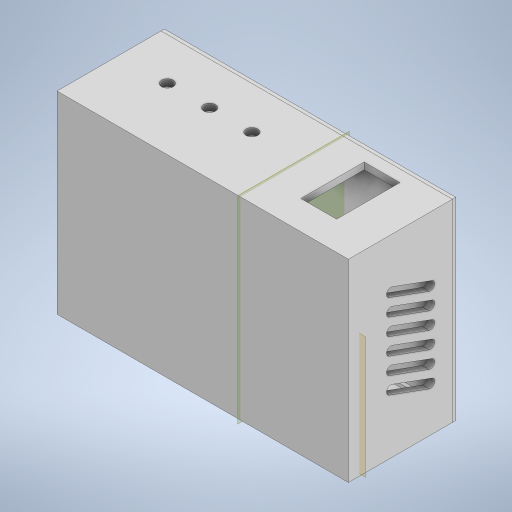
# Autodesk Inventor part: obudowa_attocube
Saved by Autodesk Inventor 2024 (Build 280153000, 153)
## iProperties
Created: 2025-11-29
Part Number: obudowa_attocube
Material: Generic
Document SubType Name: Modeling
Designer: tkazi
Density: 1 g/cm^3
Appearance: Default
Author: tkazi
Autodesk Inventor part; units mm, degrees
ref_plane "YZ Plane" through (0, 0, 0) normal (1, 0, 0) x (0, 1, 0)
ref_plane "XZ Plane" through (0, 0, 0) normal (0, 1, 0) x (-1, 0, 0)
ref_plane "XY Plane" through (0, 0, 0) normal (0, 0, 1) x (1, 0, 0)
ref_plane "Work Plane1" through (0, 0, 0) normal (0, 0, 1) x (1, 0, 0)
sketch "Sketch1" plane through (0, 0, 0) normal (0, 0, 1) x (1, 0, 0)
  line L0 (-218.6, -123.6) -> (-55.2, -123.6) projected
  line L1 (-55.2, -123.6) -> (-55.2, -58.2) projected
  line L2 (-55.2, -58.2) -> (-218.6, -58.2) projected
  line L3 (-218.6, -58.2) -> (-218.6, -123.6) projected
  circle A0 centre (-61.32, -115.13) radius 1.005 projected
  circle A1 centre (-71.48, -115.13) radius 1.005 projected
  circle A2 centre (-81.8, -118.4) radius 1.6 projected
  circle A3 centre (-91.52, -115.13) radius 1.005 projected
  circle A4 centre (-66.4, -110.05) radius 0.445 projected
  circle A5 centre (-68.94, -110.05) radius 0.445 projected
  circle A6 centre (-77.08, -109.65) radius 0.55 projected
  circle A7 centre (-77.08, -107.11) radius 0.55 projected
  circle A8 centre (-96.6, -110.05) radius 0.445 projected
  circle A9 centre (-99.14, -110.05) radius 0.445 projected
  circle A10 centre (-101.68, -115.13) radius 1.005 projected
  circle A11 centre (-121.72, -115.13) radius 1.005 projected
  circle A12 centre (-131.88, -115.13) radius 1.005 projected
  circle A13 centre (-107.28, -109.65) radius 0.55 projected
  circle A14 centre (-107.28, -107.11) radius 0.55 projected
  circle A15 centre (-126.8, -110.05) radius 0.445 projected
  circle A16 centre (-129.34, -110.05) radius 0.445 projected
  circle A17 centre (-137.48, -109.65) radius 0.55 projected
  circle A18 centre (-137.48, -107.11) radius 0.55 projected
  circle A19 centre (-77.08, -104.57) radius 0.55 projected
  circle A20 centre (-77.08, -96.83) radius 0.55 projected
  circle A21 centre (-77.08, -94.29) radius 0.55 projected
  circle A22 centre (-77.08, -91.75) radius 0.55 projected
  circle A23 centre (-107.28, -104.57) radius 0.55 projected
  circle A24 centre (-137.48, -104.57) radius 0.55 projected
  circle A25 centre (-107.28, -96.83) radius 0.55 projected
  circle A26 centre (-107.28, -94.29) radius 0.55 projected
  circle A27 centre (-107.28, -91.75) radius 0.55 projected
  circle A28 centre (-137.48, -96.83) radius 0.55 projected
  circle A29 centre (-137.48, -94.29) radius 0.55 projected
  circle A30 centre (-137.48, -91.75) radius 0.55 projected
  circle A31 centre (-159.11, -115.13) radius 0.51 projected
  circle A32 centre (-165.275, -115) radius 0.9 projected
  circle A33 centre (-170.725, -115) radius 0.9 projected
  circle A34 centre (-176.89, -115.13) radius 0.51 projected
  circle A35 centre (-159.11, -112.59) radius 0.51 projected
  circle A36 centre (-165.575, -111.97) radius 0.75 projected
  circle A37 centre (-159.11, -110.05) radius 0.51 projected
  circle A38 centre (-170.425, -111.97) radius 0.75 projected
  circle A39 centre (-176.89, -112.59) radius 0.51 projected
  circle A40 centre (-176.89, -110.05) radius 0.51 projected
  circle A41 centre (-159.11, -107.51) radius 0.51 projected
  circle A42 centre (-176.89, -107.51) radius 0.51 projected
  circle A43 centre (-190.29, -115.61) radius 0.4 projected
  circle A44 centre (-195.29, -115.61) radius 0.4 projected
  circle A45 centre (-203.8, -119.8) radius 0.8 projected
  arc A46 (-199.8, -118.55) -> (-198.8, -118.55) centre (-199.3, -118.55) ccw projected
  line L4 (-199.8, -117.05) -> (-199.8, -118.55) projected
  arc A47 (-198.8, -117.05) -> (-199.8, -117.05) centre (-199.3, -117.05) ccw projected
  line L5 (-198.8, -118.55) -> (-198.8, -117.05) projected
  arc A48 (-208.8, -118.55) -> (-207.8, -118.55) centre (-208.3, -118.55) ccw projected
  line L6 (-208.8, -117.05) -> (-208.8, -118.55) projected
  arc A49 (-207.8, -117.05) -> (-208.8, -117.05) centre (-208.3, -117.05) ccw projected
  line L7 (-207.8, -118.55) -> (-207.8, -117.05) projected
  arc A50 (-204.45, -116.3) -> (-204.45, -117.3) centre (-204.45, -116.8) ccw projected
  line L8 (-203.15, -116.3) -> (-204.45, -116.3) projected
  arc A51 (-203.15, -117.3) -> (-203.15, -116.3) centre (-203.15, -116.8) ccw projected
  line L9 (-204.45, -117.3) -> (-203.15, -117.3) projected
  circle A52 centre (-214.4, -115.8) radius 1.6 projected
  circle A53 centre (-188.555, -108.845) radius 0.55 projected
  circle A54 centre (-191.095, -108.845) radius 0.55 projected
  circle A55 centre (-193.635, -108.845) radius 0.55 projected
  arc A56 (-204.8, -110.3) -> (-204.8, -111.3) centre (-204.8, -110.8) ccw projected
  line L10 (-202.8, -110.3) -> (-204.8, -110.3) projected
  arc A57 (-202.8, -111.3) -> (-202.8, -110.3) centre (-202.8, -110.8) ccw projected
  line L11 (-204.8, -111.3) -> (-202.8, -111.3) projected
  circle A58 centre (-214.2, -109.2) radius 0.3 projected
  circle A59 centre (-159.11, -104.97) radius 0.51 projected
  circle A60 centre (-176.89, -104.97) radius 0.51 projected
  circle A61 centre (-159.11, -102.43) radius 0.51 projected
  circle A62 centre (-159.11, -99.89) radius 0.51 projected
  circle A63 centre (-176.89, -102.43) radius 0.51 projected
  circle A64 centre (-176.89, -99.89) radius 0.51 projected
  circle A65 centre (-159.11, -97.35) radius 0.51 projected
  circle A66 centre (-176.89, -97.35) radius 0.51 projected
  circle A67 centre (-159.11, -94.81) radius 0.51 projected
  circle A68 centre (-159.11, -92.27) radius 0.51 projected
  circle A69 centre (-176.89, -94.81) radius 0.51 projected
  circle A70 centre (-176.89, -92.27) radius 0.51 projected
  circle A71 centre (-188.5, -101.8) radius 0.4 projected
  circle A72 centre (-193.5, -101.8) radius 0.4 projected
  circle A73 centre (-199.4, -105.4) radius 0.3 projected
  circle A74 centre (-203, -105.4) radius 0.3 projected
  circle A75 centre (-206.4, -105.4) radius 0.3 projected
  circle A76 centre (-210, -105.4) radius 0.3 projected
  circle A77 centre (-214.2, -105.6) radius 0.3 projected
  circle A78 centre (-187.12, -92.4) radius 0.5 projected
  circle A79 centre (-189.66, -92.4) radius 0.5 projected
  circle A80 centre (-192.2, -92.4) radius 0.5 projected
  circle A81 centre (-63.7636, -91.4753) radius 0.4 projected
  circle A82 centre (-65.7635, -91.4753) radius 0.4 projected
  circle A83 centre (-93.9635, -91.4753) radius 0.4 projected
  circle A84 centre (-95.9636, -91.4753) radius 0.4 projected
  circle A85 centre (-77.08, -84.01) radius 0.55 projected
  circle A86 centre (-77.08, -81.47) radius 0.55 projected
  circle A87 centre (-77.08, -78.93) radius 0.55 projected
  circle A88 centre (-124.1636, -91.4753) radius 0.4 projected
  circle A89 centre (-126.1636, -91.4753) radius 0.4 projected
  circle A90 centre (-107.28, -84.01) radius 0.55 projected
  circle A91 centre (-107.28, -81.47) radius 0.55 projected
  circle A92 centre (-107.28, -78.93) radius 0.55 projected
  circle A93 centre (-137.48, -84.01) radius 0.55 projected
  circle A94 centre (-137.48, -81.47) radius 0.55 projected
  circle A95 centre (-137.48, -78.93) radius 0.55 projected
  circle A96 centre (-77.08, -71.19) radius 0.55 projected
  circle A97 centre (-64.91, -67.39) radius 0.4 projected
  circle A98 centre (-66.91, -67.39) radius 0.4 projected
  circle A99 centre (-77.08, -68.65) radius 0.55 projected
  circle A100 centre (-77.08, -66.11) radius 0.55 projected
  circle A101 centre (-95.11, -67.39) radius 0.4 projected
  circle A102 centre (-97.11, -67.39) radius 0.4 projected
  circle A103 centre (-107.28, -71.19) radius 0.55 projected
  circle A104 centre (-137.48, -71.19) radius 0.55 projected
  circle A105 centre (-107.28, -68.65) radius 0.55 projected
  circle A106 centre (-107.28, -66.11) radius 0.55 projected
  circle A107 centre (-117, -64.2) radius 1.6 projected
  circle A108 centre (-125.31, -67.39) radius 0.4 projected
  circle A109 centre (-127.31, -67.39) radius 0.4 projected
  circle A110 centre (-137.48, -68.65) radius 0.55 projected
  circle A111 centre (-137.48, -66.11) radius 0.55 projected
  circle A112 centre (-159.11, -89.73) radius 0.51 projected
  circle A113 centre (-176.89, -89.73) radius 0.51 projected
  circle A114 centre (-159.11, -87.19) radius 0.51 projected
  circle A115 centre (-159.11, -84.65) radius 0.51 projected
  circle A116 centre (-176.89, -87.19) radius 0.51 projected
  circle A117 centre (-176.89, -84.65) radius 0.51 projected
  circle A118 centre (-159.11, -82.11) radius 0.51 projected
  circle A119 centre (-176.89, -82.11) radius 0.51 projected
  circle A120 centre (-159.11, -79.57) radius 0.51 projected
  circle A121 centre (-176.89, -79.57) radius 0.51 projected
  circle A122 centre (-187.26, -86.8) radius 0.5 projected
  circle A123 centre (-189.8, -86.8) radius 0.5 projected
  circle A124 centre (-192.34, -86.8) radius 0.5 projected
  circle A125 centre (-185.8, -78.8) radius 0.5 projected
  circle A126 centre (-159.11, -77.03) radius 0.51 projected
  circle A127 centre (-159.11, -74.49) radius 0.51 projected
  circle A128 centre (-176.89, -77.03) radius 0.51 projected
  circle A129 centre (-176.89, -74.49) radius 0.51 projected
  circle A130 centre (-159.11, -71.95) radius 0.51 projected
  circle A131 centre (-176.89, -71.95) radius 0.51 projected
  circle A132 centre (-159.11, -69.41) radius 0.51 projected
  circle A133 centre (-159.11, -66.87) radius 0.51 projected
  circle A134 centre (-165.46, -67.1) radius 0.51 projected
  circle A135 centre (-176.89, -69.41) radius 0.51 projected
  circle A136 centre (-168, -67.1) radius 0.51 projected
  circle A137 centre (-170.54, -67.1) radius 0.51 projected
  circle A138 centre (-176.89, -66.87) radius 0.51 projected
  circle A139 centre (-185.8, -76.26) radius 0.5 projected
  circle A140 centre (-185.8, -73.72) radius 0.5 projected
  circle A141 centre (-192.75, -66.375) radius 0.4 projected
  circle A142 centre (-192.75, -64.375) radius 0.4 projected
  circle A143 centre (-117, -64.2) radius 1.35
  circle A144 centre (-214.4, -115.8) radius 1.35
  circle A145 centre (-81.8, -118.4) radius 1.35
  circle A146 centre (-214.4, -115.8) radius 4
  circle A147 centre (-117, -64.2) radius 4
  circle A148 centre (-81.8, -118.4) radius 4
  point P0 (0, 0)
  dimension "d0" = 2.7
  dimension "d1" = 2.7
  dimension "d2" = 2.7
  dimension "d3" = 8
  dimension "d4" = 8
  dimension "d5" = 8
  constraints: 6 centre point, 6 coincident
  measures "d0" diameter of A143
  measures "d1" diameter of A144
  measures "d2" diameter of A145
  measures "d3" diameter of A147
  measures "d4" diameter of A148
  measures "d5" diameter of A146
extrude "Extrusion1" add sketch "Sketch1" along normal blind 5 contours A2 | A52 | A107 | A146 | A147 | A148
sketch "Sketch2" plane through (-81.8, -118.4, 5) normal (0, 0, 1) x (1, 0, 0)
  line L0 (-136.8, -5.2) -> (26.6, -5.2) projected
  line L1 (-136.8, 60.2) -> (-136.8, -5.2) projected
  line L2 (26.6, 60.2) -> (-136.8, 60.2) projected
  line L3 (26.6, -5.2) -> (26.6, 60.2) projected
  circle A0 centre (20.48, 3.27) radius 1.005 projected
  circle A1 centre (10.32, 3.27) radius 1.005 projected
  circle A2 centre (0, 0) radius 1.6 projected
  circle A3 centre (-9.72, 3.27) radius 1.005 projected
  circle A4 centre (15.4, 8.35) radius 0.445 projected
  circle A5 centre (12.86, 8.35) radius 0.445 projected
  circle A6 centre (4.72, 8.75) radius 0.55 projected
  circle A7 centre (4.72, 11.29) radius 0.55 projected
  circle A8 centre (-14.8, 8.35) radius 0.445 projected
  circle A9 centre (-17.34, 8.35) radius 0.445 projected
  circle A10 centre (-19.88, 3.27) radius 1.005 projected
  circle A11 centre (-39.92, 3.27) radius 1.005 projected
  circle A12 centre (-50.08, 3.27) radius 1.005 projected
  circle A13 centre (-25.48, 8.75) radius 0.55 projected
  circle A14 centre (-25.48, 11.29) radius 0.55 projected
  circle A15 centre (-45, 8.35) radius 0.445 projected
  circle A16 centre (-47.54, 8.35) radius 0.445 projected
  circle A17 centre (-55.68, 8.75) radius 0.55 projected
  circle A18 centre (-55.68, 11.29) radius 0.55 projected
  circle A19 centre (4.72, 13.83) radius 0.55 projected
  circle A20 centre (4.72, 21.57) radius 0.55 projected
  circle A21 centre (4.72, 24.11) radius 0.55 projected
  circle A22 centre (4.72, 26.65) radius 0.55 projected
  circle A23 centre (-25.48, 13.83) radius 0.55 projected
  circle A24 centre (-55.68, 13.83) radius 0.55 projected
  circle A25 centre (-25.48, 21.57) radius 0.55 projected
  circle A26 centre (-25.48, 24.11) radius 0.55 projected
  circle A27 centre (-25.48, 26.65) radius 0.55 projected
  circle A28 centre (-55.68, 21.57) radius 0.55 projected
  circle A29 centre (-55.68, 24.11) radius 0.55 projected
  circle A30 centre (-55.68, 26.65) radius 0.55 projected
  circle A31 centre (-77.31, 3.27) radius 0.51 projected
  circle A32 centre (-83.475, 3.4) radius 0.9 projected
  circle A33 centre (-88.925, 3.4) radius 0.9 projected
  circle A34 centre (-95.09, 3.27) radius 0.51 projected
  circle A35 centre (-77.31, 5.81) radius 0.51 projected
  circle A36 centre (-83.775, 6.43) radius 0.75 projected
  circle A37 centre (-77.31, 8.35) radius 0.51 projected
  circle A38 centre (-88.625, 6.43) radius 0.75 projected
  circle A39 centre (-95.09, 5.81) radius 0.51 projected
  circle A40 centre (-95.09, 8.35) radius 0.51 projected
  circle A41 centre (-77.31, 10.89) radius 0.51 projected
  circle A42 centre (-95.09, 10.89) radius 0.51 projected
  circle A43 centre (-108.49, 2.79) radius 0.4 projected
  circle A44 centre (-113.49, 2.79) radius 0.4 projected
  circle A45 centre (-122, -1.4) radius 0.8 projected
  arc A46 (-118, -0.15) -> (-117, -0.15) centre (-117.5, -0.15) ccw projected
  line L4 (-117, -0.15) -> (-117, 1.35) projected
  arc A47 (-117, 1.35) -> (-118, 1.35) centre (-117.5, 1.35) ccw projected
  line L5 (-118, 1.35) -> (-118, -0.15) projected
  arc A48 (-127, -0.15) -> (-126, -0.15) centre (-126.5, -0.15) ccw projected
  line L6 (-126, -0.15) -> (-126, 1.35) projected
  arc A49 (-126, 1.35) -> (-127, 1.35) centre (-126.5, 1.35) ccw projected
  line L7 (-127, 1.35) -> (-127, -0.15) projected
  arc A50 (-122.65, 2.1) -> (-122.65, 1.1) centre (-122.65, 1.6) ccw projected
  line L8 (-122.65, 1.1) -> (-121.35, 1.1) projected
  arc A51 (-121.35, 1.1) -> (-121.35, 2.1) centre (-121.35, 1.6) ccw projected
  line L9 (-121.35, 2.1) -> (-122.65, 2.1) projected
  circle A52 centre (-132.6, 2.6) radius 1.6 projected
  circle A53 centre (-106.755, 9.555) radius 0.55 projected
  circle A54 centre (-109.295, 9.555) radius 0.55 projected
  circle A55 centre (-111.835, 9.555) radius 0.55 projected
  arc A56 (-123, 8.1) -> (-123, 7.1) centre (-123, 7.6) ccw projected
  line L10 (-123, 7.1) -> (-121, 7.1) projected
  arc A57 (-121, 7.1) -> (-121, 8.1) centre (-121, 7.6) ccw projected
  line L11 (-121, 8.1) -> (-123, 8.1) projected
  circle A58 centre (-132.4, 9.2) radius 0.3 projected
  circle A59 centre (-77.31, 13.43) radius 0.51 projected
  circle A60 centre (-95.09, 13.43) radius 0.51 projected
  circle A61 centre (-77.31, 15.97) radius 0.51 projected
  circle A62 centre (-77.31, 18.51) radius 0.51 projected
  circle A63 centre (-95.09, 15.97) radius 0.51 projected
  circle A64 centre (-95.09, 18.51) radius 0.51 projected
  circle A65 centre (-77.31, 21.05) radius 0.51 projected
  circle A66 centre (-95.09, 21.05) radius 0.51 projected
  circle A67 centre (-77.31, 23.59) radius 0.51 projected
  circle A68 centre (-77.31, 26.13) radius 0.51 projected
  circle A69 centre (-95.09, 23.59) radius 0.51 projected
  circle A70 centre (-95.09, 26.13) radius 0.51 projected
  circle A71 centre (-106.7, 16.6) radius 0.4 projected
  circle A72 centre (-111.7, 16.6) radius 0.4 projected
  circle A73 centre (-117.6, 13) radius 0.3 projected
  circle A74 centre (-121.2, 13) radius 0.3 projected
  circle A75 centre (-124.6, 13) radius 0.3 projected
  circle A76 centre (-128.2, 13) radius 0.3 projected
  circle A77 centre (-132.4, 12.8) radius 0.3 projected
  circle A78 centre (-105.32, 26) radius 0.5 projected
  circle A79 centre (-107.86, 26) radius 0.5 projected
  circle A80 centre (-110.4, 26) radius 0.5 projected
  circle A81 centre (18.0364, 26.9247) radius 0.4 projected
  circle A82 centre (16.0365, 26.9247) radius 0.4 projected
  circle A83 centre (-12.1636, 26.9247) radius 0.4 projected
  circle A84 centre (-14.1636, 26.9247) radius 0.4 projected
  circle A85 centre (4.72, 34.39) radius 0.55 projected
  circle A86 centre (4.72, 36.93) radius 0.55 projected
  circle A87 centre (4.72, 39.47) radius 0.55 projected
  circle A88 centre (-42.3636, 26.9247) radius 0.4 projected
  circle A89 centre (-44.3636, 26.9247) radius 0.4 projected
  circle A90 centre (-25.48, 34.39) radius 0.55 projected
  circle A91 centre (-25.48, 36.93) radius 0.55 projected
  circle A92 centre (-25.48, 39.47) radius 0.55 projected
  circle A93 centre (-55.68, 34.39) radius 0.55 projected
  circle A94 centre (-55.68, 36.93) radius 0.55 projected
  circle A95 centre (-55.68, 39.47) radius 0.55 projected
  circle A96 centre (4.72, 47.21) radius 0.55 projected
  circle A97 centre (16.89, 51.01) radius 0.4 projected
  circle A98 centre (14.89, 51.01) radius 0.4 projected
  circle A99 centre (4.72, 49.75) radius 0.55 projected
  circle A100 centre (4.72, 52.29) radius 0.55 projected
  circle A101 centre (-13.31, 51.01) radius 0.4 projected
  circle A102 centre (-15.31, 51.01) radius 0.4 projected
  circle A103 centre (-25.48, 47.21) radius 0.55 projected
  circle A104 centre (-55.68, 47.21) radius 0.55 projected
  circle A105 centre (-25.48, 49.75) radius 0.55 projected
  circle A106 centre (-25.48, 52.29) radius 0.55 projected
  circle A107 centre (-35.2, 54.2) radius 1.6 projected
  circle A108 centre (-43.51, 51.01) radius 0.4 projected
  circle A109 centre (-45.51, 51.01) radius 0.4 projected
  circle A110 centre (-55.68, 49.75) radius 0.55 projected
  circle A111 centre (-55.68, 52.29) radius 0.55 projected
  circle A112 centre (-77.31, 28.67) radius 0.51 projected
  circle A113 centre (-95.09, 28.67) radius 0.51 projected
  circle A114 centre (-77.31, 31.21) radius 0.51 projected
  circle A115 centre (-77.31, 33.75) radius 0.51 projected
  circle A116 centre (-95.09, 31.21) radius 0.51 projected
  circle A117 centre (-95.09, 33.75) radius 0.51 projected
  circle A118 centre (-77.31, 36.29) radius 0.51 projected
  circle A119 centre (-95.09, 36.29) radius 0.51 projected
  circle A120 centre (-77.31, 38.83) radius 0.51 projected
  circle A121 centre (-95.09, 38.83) radius 0.51 projected
  circle A122 centre (-105.46, 31.6) radius 0.5 projected
  circle A123 centre (-108, 31.6) radius 0.5 projected
  circle A124 centre (-110.54, 31.6) radius 0.5 projected
  circle A125 centre (-104, 39.6) radius 0.5 projected
  circle A126 centre (-77.31, 41.37) radius 0.51 projected
  circle A127 centre (-77.31, 43.91) radius 0.51 projected
  circle A128 centre (-95.09, 41.37) radius 0.51 projected
  circle A129 centre (-95.09, 43.91) radius 0.51 projected
  circle A130 centre (-77.31, 46.45) radius 0.51 projected
  circle A131 centre (-95.09, 46.45) radius 0.51 projected
  circle A132 centre (-77.31, 48.99) radius 0.51 projected
  circle A133 centre (-77.31, 51.53) radius 0.51 projected
  circle A134 centre (-83.66, 51.3) radius 0.51 projected
  circle A135 centre (-95.09, 48.99) radius 0.51 projected
  circle A136 centre (-86.2, 51.3) radius 0.51 projected
  circle A137 centre (-88.74, 51.3) radius 0.51 projected
  circle A138 centre (-95.09, 51.53) radius 0.51 projected
  circle A139 centre (-104, 42.14) radius 0.5 projected
  circle A140 centre (-104, 44.68) radius 0.5 projected
  circle A141 centre (-110.95, 52.025) radius 0.4 projected
  circle A142 centre (-110.95, 54.025) radius 0.4 projected
  line L12 (27.1, 60.7) -> (-137.3, 60.7)
  line L13 (-137.3, 60.7) -> (-137.3, -5.7)
  line L14 (-137.3, -5.7) -> (27.1, -5.7)
  line L15 (27.1, -5.7) -> (27.1, 60.7)
  line L16 (31.1, 64.7) -> (-141.3, 64.7)
  line L17 (-141.3, 64.7) -> (-141.3, -9.7)
  line L18 (-141.3, -9.7) -> (31.1, -9.7)
  line L19 (31.1, -9.7) -> (31.1, 64.7)
  line L20 (31.1, 64.7) -> (-141.3, 64.7)
  line L21 (-141.3, 64.7) -> (-141.3, 104.7)
  line L22 (-141.3, 104.7) -> (31.1, 104.7)
  line L23 (31.1, 104.7) -> (31.1, 64.7)
  point P0 (81.8, 118.4)
  dimension "d10" = 0.5
  dimension "side_walls" = 4
  dimension "d15" = 40
  constraints: 24 end point, 3 parallel, 1 perpendicular, 6 other
  measures "d10" distance between parallel lines of L3 L15
  measures "side_walls" distance between parallel lines of L15 L19
  measures "d15" distance of L16.end L21.end
extrude "Extrusion2" add sketch "Sketch2" along normal blind 1.5 contours L1 L2 L3 L0 | A0 | A1 | A2 | A3 | A4 | A5 | A6 | A7 | A8 | A9 | A10 | A11 | A12 | A13 | A14 | A15 | A16 | A17 | A18 | A19 | A20 | A21 | A22 | A23 | A24 | A25 | A26 | A27 | A28 | A29 | A30 | A31 | A32 | A33 | A34 | A35 | A36 | A37 | A38 | A39 | A40 | A41 | A42 | A43 | A44 | A45 | L5 A47 L4 A46 | L7 A49 L6 A48 | L9 A51 L8 A50 | A52 | A53 | A54 | A55 | L11 A57 L10 A56 | A58 | A59 | A60 | A61 | A62 | A63 | A64 | A65 | A66 | A67 | A68 | A69 | A70 | A71 | A72 | A73 | A74 | A75 | A76 | A77 | A78 | A79 | A80 | A81 | A82 | A83 | A84 | A85 | A86 | A87 | A88 | A89 | A90 | A91 | A92 | A93 | A94 | A95 | A96 | A97 | A98 | A99 | A100 | A101 | A102 | A103 | A104 | A105 | A106 | A107 | A108 | A109 | A110 | A111 | A112 | A113 | A114 | A115 | A116 | A117 | A118 | A119 | A120 | A121 | A122 | A123 | A124 | A125 | A126 | A127 | A128 | A129 | A130 | A131 | A132 | A133 | A134 | A135 | A136 | A137 | A138 | A139 | A140 | A141 | A142 | L15 L14 L13 L12 | L19 L18 L17 L16 | L16 L21 L22 L23
sketch "Sketch3" plane through (-81.8, -118.4, 5) normal (0, 0, -1) x (-1, 0, 0)
  line L0 (141.3, -9.7) -> (-31.1, -9.7) projected
  line L1 (141.3, 104.7) -> (141.3, -9.7) projected
  line L2 (-31.1, -9.7) -> (-31.1, 104.7) projected
  line L3 (-31.1, 104.7) -> (141.3, 104.7) projected
  line L4 (-27.1, 100.7) -> (-27.1, -5.7)
  line L5 (-27.1, -5.7) -> (137.3, -5.7)
  line L6 (137.3, -5.7) -> (137.3, 100.7)
  line L7 (137.3, 100.7) -> (-27.1, 100.7)
  point P0 (-81.8, 118.4)
  dimension "d16" = 4
  constraints: 8 end point, 3 other
  measures "d16" distance between parallel lines of L2 L4
extrude "Extrusion3" add sketch "Sketch3" along normal blind 60
sketch "Sketch4" plane through (-223.1, -13.7, 6.5) normal (0, 1, 0) x (1, 0, 0)
  line L0 (127.2, 54.5) -> (148.4, 54.5)
  line L1 (148.4, 54.5) -> (148.4, 17)
  line L2 (148.4, 17) -> (127.2, 17)
  line L3 (127.2, 17) -> (127.2, 54.5)
  circle A0 centre (28.7575, 36.5) radius 3.425
  circle A1 centre (53.7575, 36.5) radius 3.425
  circle A2 centre (78.7575, 36.5) radius 3.425
  line L4 (0, 0) -> (0, 61.5) projected
  line L5 (172.4, 0) -> (0, 0) projected
  line L6 (172.4, 61.5) -> (172.4, 0) projected
  line L7 (0, 61.5) -> (172.4, 61.5) projected
  line L8 (168.4, 1.5) -> (168.4, 61.5) projected
  point P0 (223.1, 6.5)
  dimension "d17" = 37.5
  dimension "d18" = 21.2
  dimension "d19" = 6.85
  dimension "d22" = 25
  dimension "d27" = 7
  dimension "d28" = 20
  dimension "d31" = 25
  constraints: 8 end point, 3 centre point, 2 horizontal, 2 parallel, 1 perpendicular, 4 other
  measures "d17" distance of L0.end L1.end
  measures "d18" distance of L1.end L2.end
  measures "d19" diameter of A0
  measures "d22" distance of A0.centre A1.centre
  measures "d27" distance between parallel lines of L7 L0
  measures "d28" distance between parallel lines of L8 L1
  measures "d31" distance from line of L7 A1.centre
extrude "Extrusion4" cut sketch "Sketch4" against normal blind 60 contours L0 L1 L2 L3 | A0 | A1 | A2
sketch "Sketch5" plane through (-223.1, -128.1, 6.5) normal (0, -1, 0) x (1, 0, 0)
  circle A0 centre (156.7, -15.195) radius 0.8 projected
  circle A1 centre (126.5, -15.195) radius 0.8 projected
  circle A2 centre (19.3, -13.095) radius 3.25 projected
  circle A3 centre (19.3, -13.095) radius 4
  circle A4 centre (156.7, -15.195) radius 6.35
  circle A5 centre (126.5, -15.195) radius 6.35
  circle A6 centre (96.3, -15.195) radius 6.35
  point P0 (223.1, -6.5)
  dimension "d32" = 8
  dimension "d33" = 12.7
  dimension "d34" = 12.7
  dimension "d35" = 12.7
  dimension "d36" = 30.2
  constraints: 4 centre point, 3 coincident, 1 horizontal alignment
  measures "d32" diameter of A3
  measures "d33" diameter of A4
  measures "d34" diameter of A5
  measures "d35" diameter of A6
  measures "d36" distance of A6.centre A1.centre
extrude "Extrusion5" cut sketch "Sketch5" against normal blind 60 contours A0 | A1 | A2 | A3 | A4 | A5 | A6
sketch "Sketch6" plane through (-50.7, -128.1, 6.5) normal (1, 0, 0) x (0, 0, -1)
  line L0 (61.5, 114.4) -> (0, 114.4) projected
  line L1 (0, 0) -> (0, 114.4) projected
  line L2 (61.5, 0) -> (0, 0) projected
  line L3 (61.5, 114.4) -> (61.5, 0) projected
  line L4 (25.0218, 85.022) -> (48.5141, 76.4715) construction
  line L5 (24.1667, 82.6727) -> (47.659, 74.1222)
  line L6 (49.3691, 78.8207) -> (25.8768, 87.3712)
  arc A0 (25.8768, 87.3712) -> (24.1667, 82.6727) centre (25.0218, 85.022) ccw
  arc A1 (47.659, 74.1222) -> (49.3691, 78.8207) centre (48.5141, 76.4715) ccw
  line L7 (25.0218, 85.022) -> (50.0218, 85.022) construction
  line L8 (49.3691, 68.8207) -> (25.8768, 77.3712)
  arc A2 (47.659, 64.1222) -> (49.3691, 68.8207) centre (48.5141, 66.4715) ccw
  line L9 (24.1667, 72.6727) -> (47.659, 64.1222)
  arc A3 (25.8768, 77.3712) -> (24.1667, 72.6727) centre (25.0218, 75.022) ccw
  line L10 (49.3691, 58.8207) -> (25.8768, 67.3712)
  arc A4 (47.659, 54.1222) -> (49.3691, 58.8207) centre (48.5141, 56.4715) ccw
  line L11 (24.1667, 62.6727) -> (47.659, 54.1222)
  arc A5 (25.8768, 67.3712) -> (24.1667, 62.6727) centre (25.0218, 65.022) ccw
  line L12 (49.3691, 48.8207) -> (25.8768, 57.3712)
  arc A6 (47.659, 44.1222) -> (49.3691, 48.8207) centre (48.5141, 46.4715) ccw
  line L13 (24.1667, 52.6727) -> (47.659, 44.1222)
  arc A7 (25.8768, 57.3712) -> (24.1667, 52.6727) centre (25.0218, 55.022) ccw
  line L14 (49.3691, 38.8207) -> (25.8768, 47.3712)
  arc A8 (47.659, 34.1222) -> (49.3691, 38.8207) centre (48.5141, 36.4715) ccw
  line L15 (24.1667, 42.6727) -> (47.659, 34.1222)
  arc A9 (25.8768, 47.3712) -> (24.1667, 42.6727) centre (25.0218, 45.022) ccw
  line L16 (49.3691, 28.8207) -> (25.8768, 37.3712)
  arc A10 (47.659, 24.1222) -> (49.3691, 28.8207) centre (48.5141, 26.4715) ccw
  line L17 (24.1667, 32.6727) -> (47.659, 24.1222)
  arc A11 (25.8768, 37.3712) -> (24.1667, 32.6727) centre (25.0218, 35.022) ccw
  point P0 (6.5, 128.1)
  point P1 (26.87, 49.745)
  point P2 (36.7679, 80.7467)
  dimension "d39" = 25
  dimension "d40" = 20
  dimension "d41" = 5
  dimension "d44" = 10
  constraints: 30 end point, 24 point on circle, 12 centre point, 4 tangent, 1 equal length, 1 horizontal, 1 midpoint, 1 parallel, 1 vertical, 51 other
  measures "d39" distance of L4.start L4.end
  measures "d40" angle of L4 L7
  measures "d41" diameter of A1
  measures "d44" distance of L6.start L8.start
extrude "Extrusion6" cut sketch "Sketch6" against normal through all contours A0 L6 A1 L5 | A2 L9 A3 L8 | A4 L11 A5 L10 | A6 L13 A7 L12 | A8 L15 A9 L14 | A10 L17 A11 L16
ref_plane "Work Plane2" through (-114.7, -124.1, 5) normal (-1, 0, 0) x (0, 0, 1)
sketch "Sketch11" plane through (-81.8, -118.4, -55) normal (0, 0, -1) x (-1, 0, 0)
  line L0 (141.3, 104.7) -> (-31.1, 104.7) projected
  line L1 (-31.1, 104.7) -> (-31.1, -9.7) projected
  line L2 (-31.1, -9.7) -> (141.3, -9.7) projected
  line L3 (141.3, -9.7) -> (141.3, 104.7) projected
  line L4 (-27.1, 100.7) -> (137.3, 100.7) projected
  line L5 (137.3, 100.7) -> (137.3, -5.7) projected
  line L6 (137.3, -5.7) -> (-27.1, -5.7) projected
  line L7 (-27.1, -5.7) -> (-27.1, 100.7) projected
  circle A0 centre (-27.1, -5.7) radius 5
  circle A1 centre (-27.1, 100.7) radius 5
  circle A2 centre (137.3, 100.7) radius 5
  circle A3 centre (137.3, -5.7) radius 5
  point P0 (-81.8, 118.4)
  point P1 (137.3, -0.7)
  point P2 (132.3, -5.7)
  point P3 (-22.1, -5.7)
  point P4 (-27.1, -0.7)
  point P5 (132.3, 100.7)
  point P6 (137.3, 95.7)
  point P7 (-27.1, 95.7)
  point P8 (-22.1, 100.7)
  dimension "d77" = 10
  dimension "d78" = 10
  dimension "d79" = 10
  dimension "d80" = 10
  constraints: 4 centre point, 4 coincident
  measures "d77" diameter of A0
  measures "d78" diameter of A1
  measures "d79" diameter of A2
  measures "d80" diameter of A3
extrude "Extrusion11" add sketch "Sketch11" against normal blind 10 contours L4 L5 A2 | A1 L7 L4 | L5 L6 A3 | A0 L6 L7
chamfer "Chamfer1" distance 5 angle 45 4 edges at (-215.5645, -120.5645, -45) (-215.5645, -21.2355, -45) (-58.2355, -21.2355, -45) (-58.2355, -120.5645, -45)
sketch "Sketch12" plane through (-81.8, -118.4, -55) normal (0, 0, -1) x (-1, 0, 0)
  arc A0 (-22.1, -5.7) -> (-27.1, -0.7) centre (-27.1, -5.7) ccw projected
  arc A1 (-27.1, 95.7) -> (-22.1, 100.7) centre (-27.1, 100.7) ccw projected
  arc A2 (137.3, -0.7) -> (132.3, -5.7) centre (137.3, -5.7) ccw projected
  arc A3 (132.3, 100.7) -> (137.3, 95.7) centre (137.3, 100.7) ccw projected
  point P0 (-81.8, 118.4)
hole "Hole1" at (-219.1, -124.1, -55) at (-219.1, -17.7, -55) at (-54.7, -17.7, -55) at (-54.7, -124.1, -55) direction (0, 0, 1) diameter 2.7 depth 8 tip angle 118
sketch "Sketch13" plane through (-81.8, -118.4, -55) normal (0, 0, -1) x (-1, 0, 0)
  circle A0 centre (-27.1, -5.7) radius 1.35 projected
  circle A1 centre (-27.1, 100.7) radius 1.35 projected
  circle A2 centre (137.3, 100.7) radius 1.35 projected
  circle A3 centre (137.3, -5.7) radius 1.35 projected
  line L0 (141.3, 104.7) -> (-31.1, 104.7) projected
  line L1 (-31.1, 104.7) -> (-31.1, -9.7) projected
  line L2 (-31.1, -9.7) -> (141.3, -9.7) projected
  line L3 (141.3, -9.7) -> (141.3, 104.7) projected
  line L4 (-22.1, 100.7) -> (132.3, 100.7) projected
  arc A4 (132.3, 100.7) -> (137.3, 95.7) centre (137.3, 100.7) ccw projected
  line L5 (137.3, 95.7) -> (137.3, -0.7) projected
  arc A5 (137.3, -0.7) -> (132.3, -5.7) centre (137.3, -5.7) ccw projected
  line L6 (132.3, -5.7) -> (-22.1, -5.7) projected
  arc A6 (-22.1, -5.7) -> (-27.1, -0.7) centre (-27.1, -5.7) ccw projected
  line L7 (-27.1, -0.7) -> (-27.1, 95.7) projected
  arc A7 (-27.1, 95.7) -> (-22.1, 100.7) centre (-27.1, 100.7) ccw projected
  line L8 (-26.6, 95.2228) -> (-26.6, -0.2228)
  arc A8 (-21.6228, -5.2) -> (-26.6, -0.2228) centre (-27.1, -5.7) ccw
  line L9 (-21.6228, -5.2) -> (131.8228, -5.2)
  arc A9 (136.8, -0.2228) -> (131.8228, -5.2) centre (137.3, -5.7) ccw
  line L10 (136.8, -0.2228) -> (136.8, 95.2228)
  arc A10 (131.8228, 100.2) -> (136.8, 95.2228) centre (137.3, 100.7) ccw
  line L11 (131.8228, 100.2) -> (-21.6228, 100.2)
  arc A11 (-26.6, 95.2228) -> (-21.6228, 100.2) centre (-27.1, 100.7) ccw
  line L12 (-24.6, 1.3711) -> (-24.6, 93.6289)
  arc A12 (-24.6, 93.6289) -> (-20.0289, 98.2) centre (-27.1, 100.7) ccw
  line L13 (-20.0289, 98.2) -> (130.2289, 98.2)
  arc A13 (130.2289, 98.2) -> (134.8, 93.6289) centre (137.3, 100.7) ccw
  line L14 (134.8, 93.6289) -> (134.8, 1.3711)
  arc A14 (134.8, 1.3711) -> (130.2289, -3.2) centre (137.3, -5.7) ccw
  line L15 (130.2289, -3.2) -> (-20.0289, -3.2)
  arc A15 (-20.0289, -3.2) -> (-24.6, 1.3711) centre (-27.1, -5.7) ccw
  point P0 (-81.8, 118.4)
  dimension "d93" = 0.5
  dimension "d94" = 2
  constraints: 16 end point, 16 point on circle, 8 centre point, 14 other
  measures "d93" distance between parallel lines of L7 L8
  measures "d94" distance between parallel lines of L8 L12
extrude "Extrusion12" add sketch "Sketch13" against normal blind 2 separate body contours A11 L11 A10 L10 A9 L9 A8 L8
sketch "Sketch14" plane through (-81.8, -118.4, -55) normal (0, 0, -1) x (-1, 0, 0)
  circle A0 centre (-27.1, -5.7) radius 1.35 projected
  circle A1 centre (-27.1, 100.7) radius 1.35 projected
  circle A2 centre (137.3, 100.7) radius 1.35 projected
  circle A3 centre (137.3, -5.7) radius 1.35 projected
  line L0 (141.3, 104.7) -> (-31.1, 104.7) projected
  line L1 (-31.1, 104.7) -> (-31.1, -9.7) projected
  line L2 (-31.1, -9.7) -> (141.3, -9.7) projected
  line L3 (141.3, -9.7) -> (141.3, 104.7) projected
  line L4 (-22.1, 100.7) -> (132.3, 100.7) projected
  arc A4 (132.3, 100.7) -> (137.3, 95.7) centre (137.3, 100.7) ccw projected
  line L5 (137.3, 95.7) -> (137.3, -0.7) projected
  arc A5 (137.3, -0.7) -> (132.3, -5.7) centre (137.3, -5.7) ccw projected
  line L6 (132.3, -5.7) -> (-22.1, -5.7) projected
  arc A6 (-22.1, -5.7) -> (-27.1, -0.7) centre (-27.1, -5.7) ccw projected
  line L7 (-27.1, -0.7) -> (-27.1, 95.7) projected
  arc A7 (-27.1, 95.7) -> (-22.1, 100.7) centre (-27.1, 100.7) ccw projected
  point P0 (-81.8, 118.4)
extrude "Extrusion13" add sketch "Sketch14" along normal blind 2 contours A0 | A1 | A2 | A3 | L3 L2 L1 L0 | L4 A4 L5 A5 L6 A6 L7 A7 bodies 2
sketch "Sketch15" plane through (-81.8, -118.4, -57) normal (0, 0, -1) x (-1, 0, 0)
  circle A0 centre (-27.1, 100.7) radius 1.35 projected
  circle A1 centre (-27.1, -5.7) radius 1.35 projected
  circle A2 centre (137.3, 100.7) radius 1.35 projected
  circle A3 centre (137.3, -5.7) radius 1.35 projected
  point P0 (-81.8, 118.4)
hole "Hole2" at (-219.1, -124.1, -57) at (-219.1, -17.7, -57) at (-54.7, -17.7, -57) at (-54.7, -124.1, -57) direction (0, 0, 1) diameter 3.2 depth 8 tip angle 118 countersink diameter 5.6 countersink angle 90 bodies 2
equation "\"d16\" = side_walls"
body "Solid1"
